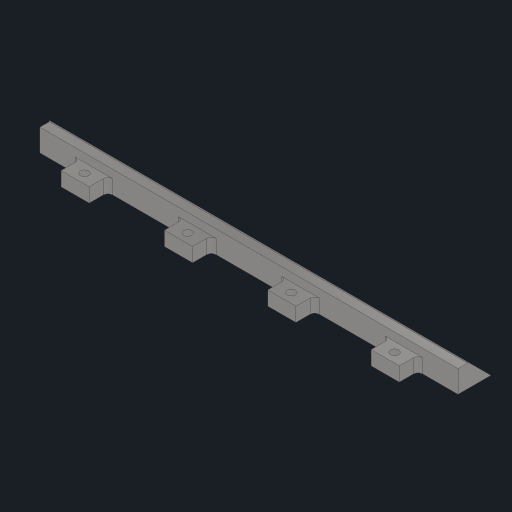
# Autodesk Inventor part: plog
Saved by Autodesk Inventor 2023 (Build 270158000, 158)
## iProperties
Created: 2024-04-10
Part Number: plog
Material: Steel, Alloy
Document SubType Name: Modeling
Designer: szymo
Density: 7.73 g/cm^3
Appearance: Semi-Polished
Mass: 140.636 g
Surface Area: 91.3762 cm^2
Volume: 18.1935 cm^3
Author: szymo
Autodesk Inventor part; units mm, degrees
ref_plane "YZ Plane" through (0, 0, 0) normal (1, 0, 0) x (0, 1, 0)
ref_plane "XZ Plane" through (0, 0, 0) normal (0, 1, 0) x (-1, 0, 0)
ref_plane "XY Plane" through (0, 0, 0) normal (0, 0, 1) x (1, 0, 0)
sketch "Sketch3" plane through (0, 0, 0) normal (1, 0, 0) x (0, 1, 0)
  line L0 (0, 0) -> (10, 0)
  line L1 (10, 0) -> (10, -10)
  line L2 (10, -10) -> (0, -10)
  line L3 (0, -10) -> (0, 0)
  line L4 (10, 0) -> (0, -10)
  line L5 (6, 0) -> (0, 0)
  line L6 (0, 0) -> (0, 12)
  line L7 (0, 12) -> (6, 12)
  line L8 (6, 12) -> (6, 0)
  line L9 (9.5, 0) -> (6, 0)
  line L10 (6, 0) -> (6, 4)
  line L11 (6, 4) -> (9.5, 4)
  line L12 (9.5, 4) -> (9.5, 0)
  dimension "d28" = 10
  dimension "d29" = 45
  dimension "d30" = 12
  dimension "d31" = 6
  dimension "d63" = 10
  dimension "d74" = 0.5
  dimension "d75" = 4
  dimension "d76" = 3.5
  constraints: 26 end point, 6 parallel, 4 point on line, 3 horizontal, 3 perpendicular
  measures "d28" distance of L0.end L1.end
  measures "d29" angle of L2 L4
  measures "d30" distance of L5.end L6.end
  measures "d31" distance of L6.end L7.end
  measures "d63" distance of L1.end L2.end
  measures "d74" distance between parallel lines of L1 L12
  measures "d75" distance between parallel lines of L11 L0
  measures "d76" distance of L10.end L11.end
extrude "Extrusion2" add sketch "Sketch3" along normal blind 178 contours L6 L7 L8 L0 | L0 L4 L3 | L8 L11 L12 L0
sketch "Sketch10" plane through (0, 0, -10) normal (0, -1, 0) x (1, 0, 0)
  line L0 (0, 14) -> (0, 22) projected
  line L1 (0, 22) -> (178, 22) projected
  line L2 (178, 14) -> (178, 22) projected
  line L3 (0, 14) -> (178, 14) projected
  line L4 (0, 10) -> (0, 14) projected
  line L5 (0, 14) -> (17, 14)
  line L6 (17, 14) -> (17, 22)
  line L7 (17, 22) -> (0, 22)
  line L8 (0, 22) -> (0, 14)
  line L9 (0, 14) -> (178, 14) projected
  line L10 (178, 22) -> (161, 22)
  line L11 (161, 22) -> (161, 14)
  line L12 (161, 14) -> (178, 14)
  line L13 (178, 14) -> (178, 22)
  line L14 (17, 22) -> (29, 22)
  line L15 (29, 22) -> (29, 14)
  line L16 (29, 14) -> (17, 14)
  line L17 (17, 14) -> (17, 22)
  line L18 (61, 22) -> (73, 22)
  line L19 (73, 22) -> (73, 14)
  line L20 (73, 14) -> (61, 14)
  line L21 (61, 14) -> (61, 22)
  line L22 (105, 22) -> (117, 22)
  line L23 (117, 22) -> (117, 14)
  line L24 (117, 14) -> (105, 14)
  line L25 (105, 14) -> (105, 22)
  line L26 (149, 22) -> (161, 22)
  line L27 (161, 22) -> (161, 14)
  line L28 (161, 14) -> (149, 14)
  line L29 (149, 14) -> (149, 22)
  line L30 (17, 22) -> (29, 14)
  line L31 (29, 22) -> (17, 14)
  line L32 (61, 22) -> (73, 14)
  line L33 (73, 22) -> (61, 14)
  line L34 (105, 22) -> (117, 14)
  line L35 (117, 22) -> (105, 14)
  line L36 (149, 22) -> (161, 14)
  line L37 (161, 22) -> (149, 14)
  point P0 (23, 18)
  point P1 (67, 18)
  point P2 (111, 18)
  point P3 (155, 18)
  dimension "d118" = 17
  dimension "d119" = 17
  dimension "d120" = 12
  dimension "d121" = 12
  dimension "d122" = 12
  dimension "d123" = 12
  dimension "d124" = 0
  dimension "d125" = 0
  dimension "d126" = 32
  dimension "d129" = 32
  dimension "d130" = 32
  constraints: 64 end point, 12 parallel, 10 point on line, 6 horizontal, 6 perpendicular, 4 midpoint
  measures "d118" distance of L7.end L6.end
  measures "d119" distance of L12.end L11.end
  measures "d120" distance of L15.end L16.end
  measures "d121" distance of L19.end L20.end
  measures "d122" distance of L23.end L24.end
  measures "d123" distance of L27.end L28.end
  measures "d124" distance between parallel lines of L6 L17
  measures "d125" distance between parallel lines of L27 L11
  measures "d126" distance between parallel lines of L23 L29
  measures "d129" distance between parallel lines of L15 L21
  measures "d130" distance between parallel lines of L19 L25
extrude "Extrusion5" cut sketch "Sketch10" against normal up to next contours L0 L1 L6 L3 | L15 L1 L21 L3 | L19 L1 L25 L3 | L23 L1 L29 L3 | L11 L1 L2 L3
hole "Hole4" at (23, 0, 8) at (67, 0, 8) at (111, 0, 8) at (155, 0, 8) direction (0, 1, 0) diameter 3.6 end through all countersink diameter 6.5 countersink angle 90 clearance for "Countersunk Flat Head Screw ISO 2009/7046" size "M3" standard "ISO"
fillet "Fillet2" radius 2 8 edges at (17, 3, 4) (29, 3, 4) (61, 3, 4) (73, 3, 4) (105, 3, 4) (117, 3, 4) (149, 3, 4) (161, 3, 4)
equation "\"d126\" = d130"
equation "\"d129\" = d130"
body "Solid2"
